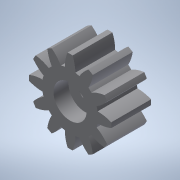
# Autodesk Inventor part: small-gear
Saved by Autodesk Inventor 2020 (Build 240168000, 168)
## iProperties
Created: 2020-05-22
Part Number: small-gear
Material: Ogólny
Document SubType Name: Modeling
Designer: blep
Density: 1 g/cm^3
Appearance: Domyślna
Author: blep
Autodesk Inventor part; units mm, degrees
ref_plane "YZ Plane" through (0, 0, 0) normal (1, 0, 0) x (0, 1, 0)
ref_plane "XZ Plane" through (0, 0, 0) normal (0, 1, 0) x (-1, 0, 0)
ref_plane "XY Plane" through (0, 0, 0) normal (0, 0, 1) x (1, 0, 0)
sketch "Szkic1" plane through (0, 0, 0) normal (0, 0, 1) x (1, 0, 0)
  arc A0 (-1.732, -4.0613) -> (-1.6613, -4.132) centre (0, -2.4) ccw projected
  arc A1 (0.05, -0.4006) -> (-0.05, -0.4006) centre (0, -2.4) ccw projected
  arc A2 (-0.05, -0.4006) -> (-0.5703, -0.483) centre (0, -2.4) ccw projected
  arc A3 (-0.5703, -0.483) -> (-0.6654, -0.5139) centre (0, -2.4) ccw projected
  arc A4 (-0.6654, -0.5139) -> (-1.1348, -0.7531) centre (0, -2.4) ccw projected
  arc A5 (-1.1348, -0.7531) -> (-1.2157, -0.8119) centre (0, -2.4) ccw projected
  arc A6 (-1.2157, -0.8119) -> (-1.5881, -1.1843) centre (0, -2.4) ccw projected
  arc A7 (-1.5881, -1.1843) -> (-1.6469, -1.2652) centre (0, -2.4) ccw projected
  arc A8 (-1.6469, -1.2652) -> (-1.8861, -1.7346) centre (0, -2.4) ccw projected
  arc A9 (-1.8861, -1.7346) -> (-1.917, -1.8297) centre (0, -2.4) ccw projected
  arc A10 (-1.917, -1.8297) -> (-1.9994, -2.35) centre (0, -2.4) ccw projected
  arc A11 (-1.9994, -2.35) -> (-1.9994, -2.45) centre (0, -2.4) ccw projected
  arc A12 (-1.9994, -2.45) -> (-1.917, -2.9703) centre (0, -2.4) ccw projected
  arc A13 (-1.917, -2.9703) -> (-1.8861, -3.0654) centre (0, -2.4) ccw projected
  arc A14 (-1.8861, -3.0654) -> (-1.6469, -3.5348) centre (0, -2.4) ccw projected
  arc A15 (-1.6469, -3.5348) -> (-1.5881, -3.6157) centre (0, -2.4) ccw projected
  arc A16 (-1.5881, -3.6157) -> (-1.2157, -3.9881) centre (0, -2.4) ccw projected
  arc A17 (-1.2157, -3.9881) -> (-1.1348, -4.0469) centre (0, -2.4) ccw projected
  arc A18 (-1.1348, -4.0469) -> (-0.6654, -4.2861) centre (0, -2.4) ccw projected
  arc A19 (-0.6654, -4.2861) -> (-0.5703, -4.317) centre (0, -2.4) ccw projected
  arc A20 (-0.5703, -4.317) -> (-0.05, -4.3994) centre (0, -2.4) ccw projected
  arc A21 (-0.05, -4.3994) -> (0.05, -4.3994) centre (0, -2.4) ccw projected
  arc A22 (0.05, -4.3994) -> (0.5703, -4.317) centre (0, -2.4) ccw projected
  arc A23 (0.5703, -4.317) -> (0.6654, -4.2861) centre (0, -2.4) ccw projected
  arc A24 (0.6654, -4.2861) -> (1.1348, -4.0469) centre (0, -2.4) ccw projected
  arc A25 (1.1348, -4.0469) -> (1.2157, -3.9881) centre (0, -2.4) ccw projected
  arc A26 (1.2157, -3.9881) -> (1.5881, -3.6157) centre (0, -2.4) ccw projected
  arc A27 (1.5881, -3.6157) -> (1.6469, -3.5348) centre (0, -2.4) ccw projected
  arc A28 (1.6469, -3.5348) -> (1.8861, -3.0654) centre (0, -2.4) ccw projected
  arc A29 (1.8861, -3.0654) -> (1.917, -2.9703) centre (0, -2.4) ccw projected
  arc A30 (1.917, -2.9703) -> (1.9994, -2.45) centre (0, -2.4) ccw projected
  arc A31 (1.9994, -2.45) -> (1.9994, -2.35) centre (0, -2.4) ccw projected
  arc A32 (1.9994, -2.35) -> (1.917, -1.8297) centre (0, -2.4) ccw projected
  arc A33 (1.917, -1.8297) -> (1.8861, -1.7346) centre (0, -2.4) ccw projected
  arc A34 (1.8861, -1.7346) -> (1.6469, -1.2652) centre (0, -2.4) ccw projected
  arc A35 (1.6469, -1.2652) -> (1.5881, -1.1843) centre (0, -2.4) ccw projected
  arc A36 (1.5881, -1.1843) -> (1.2157, -0.8119) centre (0, -2.4) ccw projected
  arc A37 (1.2157, -0.8119) -> (1.1348, -0.7531) centre (0, -2.4) ccw projected
  arc A38 (1.1348, -0.7531) -> (0.6654, -0.5139) centre (0, -2.4) ccw projected
  arc A39 (0.6654, -0.5139) -> (0.5703, -0.483) centre (0, -2.4) ccw projected
  arc A40 (0.5703, -0.483) -> (0.05, -0.4006) centre (0, -2.4) ccw projected
  circle A41 centre (0, -2.4) radius 1.5065 projected
  circle A42 centre (0, -2.4) radius 2.4
  circle A43 centre (0, -2.4) radius 15
  circle A44 centre (0, -2.4) radius 1.0065 projected
  circle A45 centre (0, -2.4) radius 1.2565
  circle A46 centre (0, -2.4) radius 2.65
  point P0 (0, 0)
  point P1 (-1.6613, -4.132)
  point P2 (-1.732, -4.0613)
  dimension "d0" = 30
  dimension "d3" = 0.25
  dimension "d12" = 0.25
  constraints: 4 centre point, 2 coincident, 1 concentric
  measures "d0" diameter of A43
  measures "d3" radial gap between concentric circles of A44 A45
  measures "d12" radial gap between concentric circles of A42 A46
extrude "Wyciągnięcie proste1" add sketch "Szkic1" against normal blind 3 contours A43
extrude "Wyciągnięcie proste2" add sketch "Szkic1" along normal blind 1.5 contours A42 A0 | A40 A39 A38 A37 A36 A35 A34 A33 A32 A31 A30 A29 A28 A27 A26 A25 A24 A23 A22 A21 A20 A19 A18 A17 A16 A15 A14 A13 A12 A11 A10 A9 A8 A7 A6 A5 A4 A3 A2 A1 | A41 | A43 | A45 | A46
sketch "Szkic2" plane through (0, -2.4, 1.5) normal (0, 0, 1) x (1, 0, 0)
  circle A0 centre (0, 0) radius 1.0065 projected
  circle A1 centre (0, 0) radius 3
  circle A2 centre (0, 0) radius 15 projected
  point P0 (0, 2.4)
  dimension "d6" = 6
  constraints: 1 centre point, 1 coincident
  measures "d6" diameter of A1
extrude "Wyciągnięcie proste3" add sketch "Szkic2" along normal blind 2.7 contours A2
spur gear teeth "Przekładnia walcowa1" teeth 12 pitch diameter 13.5 tip diameter 15.0027 root diameter 10.2375 face width 7.6 trims to tip circle yes start plane through (0, -2.4, -3) normal (0, 0, -1) x (-1, 0, 0)
sketch "Szkic3" plane through (0, -2.4, 4.2) normal (0, 0, 1) x (1, 0, 0)
  arc A0 (-6.2371, 4.1675) -> (-6.7277, 3.3178) centre (0, 0) ccw projected
  arc A1 (-6.7277, 3.3178) -> (-4.8471, 1.6454) centre (-1.5303, 7.2689) ccw projected
  arc A2 (-4.8471, 1.6454) -> (-5.0204, 0.9986) centre (0, 0) ccw projected
  arc A3 (-5.0204, 0.9986) -> (-7.4853, 0.4906) centre (-4.9597, -5.5299) ccw projected
  arc A4 (-7.4853, 0.4906) -> (-7.4853, -0.4906) centre (0, 0) ccw projected
  arc A5 (-7.4853, -0.4906) -> (-5.0204, -0.9986) centre (-4.9597, 5.5299) ccw projected
  arc A6 (-5.0204, -0.9986) -> (-4.8471, -1.6454) centre (0, 0) ccw projected
  arc A7 (-4.8471, -1.6454) -> (-6.7277, -3.3178) centre (-1.5303, -7.2689) ccw projected
  arc A8 (-6.7277, -3.3178) -> (-6.2371, -4.1675) centre (0, 0) ccw projected
  arc A9 (-6.2371, -4.1675) -> (-3.8485, -3.375) centre (-7.0601, 2.3092) ccw projected
  arc A10 (-3.8485, -3.375) -> (-3.375, -3.8485) centre (0, 0) ccw projected
  arc A11 (-3.375, -3.8485) -> (-4.1675, -6.2371) centre (2.3092, -7.0601) ccw projected
  arc A12 (-4.1675, -6.2371) -> (-3.3178, -6.7277) centre (0, 0) ccw projected
  arc A13 (-3.3178, -6.7277) -> (-1.6454, -4.8471) centre (-7.2689, -1.5303) ccw projected
  arc A14 (-1.6454, -4.8471) -> (-0.9986, -5.0204) centre (0, 0) ccw projected
  arc A15 (-0.9986, -5.0204) -> (-0.4906, -7.4853) centre (5.5299, -4.9597) ccw projected
  arc A16 (-0.4906, -7.4853) -> (0.4906, -7.4853) centre (0, 0) ccw projected
  arc A17 (0.4906, -7.4853) -> (0.9986, -5.0204) centre (-5.5299, -4.9597) ccw projected
  arc A18 (0.9986, -5.0204) -> (1.6454, -4.8471) centre (0, 0) ccw projected
  arc A19 (1.6454, -4.8471) -> (3.3178, -6.7277) centre (7.2689, -1.5303) ccw projected
  arc A20 (3.3178, -6.7277) -> (4.1675, -6.2371) centre (0, 0) ccw projected
  arc A21 (4.1675, -6.2371) -> (3.375, -3.8485) centre (-2.3092, -7.0601) ccw projected
  arc A22 (3.375, -3.8485) -> (3.8485, -3.375) centre (0, 0) ccw projected
  arc A23 (3.8485, -3.375) -> (6.2371, -4.1675) centre (7.0601, 2.3092) ccw projected
  arc A24 (6.2371, -4.1675) -> (6.7277, -3.3178) centre (0, 0) ccw projected
  arc A25 (6.7277, -3.3178) -> (4.8471, -1.6454) centre (1.5303, -7.2689) ccw projected
  arc A26 (4.8471, -1.6454) -> (5.0204, -0.9986) centre (0, 0) ccw projected
  arc A27 (5.0204, -0.9986) -> (7.4853, -0.4906) centre (4.9597, 5.5299) ccw projected
  arc A28 (7.4853, -0.4906) -> (7.4853, 0.4906) centre (0, 0) ccw projected
  arc A29 (7.4853, 0.4906) -> (5.0204, 0.9986) centre (4.9597, -5.5299) ccw projected
  arc A30 (5.0204, 0.9986) -> (4.8471, 1.6454) centre (0, 0) ccw projected
  arc A31 (4.8471, 1.6454) -> (6.7277, 3.3178) centre (1.5303, 7.2689) ccw projected
  arc A32 (6.7277, 3.3178) -> (6.2371, 4.1675) centre (0, 0) ccw projected
  arc A33 (6.2371, 4.1675) -> (3.8485, 3.375) centre (7.0601, -2.3092) ccw projected
  arc A34 (3.8485, 3.375) -> (3.375, 3.8485) centre (0, 0) ccw projected
  arc A35 (3.375, 3.8485) -> (4.1675, 6.2371) centre (-2.3092, 7.0601) ccw projected
  arc A36 (4.1675, 6.2371) -> (3.3178, 6.7277) centre (0, 0) ccw projected
  arc A37 (3.3178, 6.7277) -> (1.6454, 4.8471) centre (7.2689, 1.5303) ccw projected
  arc A38 (1.6454, 4.8471) -> (0.9986, 5.0204) centre (0, 0) ccw projected
  arc A39 (0.9986, 5.0204) -> (0.4906, 7.4853) centre (-5.5299, 4.9597) ccw projected
  arc A40 (0.4906, 7.4853) -> (-0.4906, 7.4853) centre (0, 0) ccw projected
  arc A41 (-0.4906, 7.4853) -> (-0.9986, 5.0204) centre (5.5299, 4.9597) ccw projected
  arc A42 (-0.9986, 5.0204) -> (-1.6454, 4.8471) centre (0, 0) ccw projected
  arc A43 (-1.6454, 4.8471) -> (-3.3178, 6.7277) centre (-7.2689, 1.5303) ccw projected
  arc A44 (-3.3178, 6.7277) -> (-4.1675, 6.2371) centre (0, 0) ccw projected
  arc A45 (-4.1675, 6.2371) -> (-3.375, 3.8485) centre (2.3092, 7.0601) ccw projected
  arc A46 (-3.375, 3.8485) -> (-3.8485, 3.375) centre (0, 0) ccw projected
  arc A47 (-3.8485, 3.375) -> (-6.2371, 4.1675) centre (-7.0601, -2.3092) ccw projected
  circle A48 centre (0, 0) radius 3 projected
  arc A49 (4.1139, -6.2127) -> (3.3113, -3.8376) centre (-2.3092, -7.0601) ccw
  arc A50 (3.3234, -6.6691) -> (4.1139, -6.2127) centre (0, 0) ccw
  arc A51 (1.6678, -4.7865) -> (3.3234, -6.6691) centre (7.2689, -1.5303) ccw
  arc A52 (0.9489, -4.9791) -> (1.6678, -4.7865) centre (0, 0) ccw
  arc A53 (0.4564, -7.4373) -> (0.9489, -4.9791) centre (-5.5299, -4.9597) ccw
  arc A54 (-0.4564, -7.4373) -> (0.4564, -7.4373) centre (0, 0) ccw
  arc A55 (-0.9489, -4.9791) -> (-0.4564, -7.4373) centre (5.5299, -4.9597) ccw
  arc A56 (-1.6678, -4.7865) -> (-0.9489, -4.9791) centre (0, 0) ccw
  arc A57 (-3.3234, -6.6691) -> (-1.6678, -4.7865) centre (-7.2689, -1.5303) ccw
  arc A58 (-4.1139, -6.2127) -> (-3.3234, -6.6691) centre (0, 0) ccw
  arc A59 (-3.3113, -3.8376) -> (-4.1139, -6.2127) centre (2.3092, -7.0601) ccw
  arc A60 (-3.8376, -3.3113) -> (-3.3113, -3.8376) centre (0, 0) ccw
  arc A61 (-6.2127, -4.1139) -> (-3.8376, -3.3113) centre (-7.0601, 2.3092) ccw
  arc A62 (-6.6691, -3.3234) -> (-6.2127, -4.1139) centre (0, 0) ccw
  arc A63 (-4.7865, -1.6678) -> (-6.6691, -3.3234) centre (-1.5303, -7.2689) ccw
  arc A64 (-4.9791, -0.9489) -> (-4.7865, -1.6678) centre (0, 0) ccw
  arc A65 (-7.4373, -0.4564) -> (-4.9791, -0.9489) centre (-4.9597, 5.5299) ccw
  arc A66 (-7.4373, 0.4564) -> (-7.4373, -0.4564) centre (0, 0) ccw
  arc A67 (-4.9791, 0.9489) -> (-7.4373, 0.4564) centre (-4.9597, -5.5299) ccw
  arc A68 (-4.7865, 1.6678) -> (-4.9791, 0.9489) centre (0, 0) ccw
  arc A69 (-6.6691, 3.3234) -> (-4.7865, 1.6678) centre (-1.5303, 7.2689) ccw
  arc A70 (-6.2127, 4.1139) -> (-6.6691, 3.3234) centre (0, 0) ccw
  arc A71 (-3.8376, 3.3113) -> (-6.2127, 4.1139) centre (-7.0601, -2.3092) ccw
  arc A72 (-3.3113, 3.8376) -> (-3.8376, 3.3113) centre (0, 0) ccw
  arc A73 (-4.1139, 6.2127) -> (-3.3113, 3.8376) centre (2.3092, 7.0601) ccw
  arc A74 (-3.3234, 6.6691) -> (-4.1139, 6.2127) centre (0, 0) ccw
  arc A75 (-1.6678, 4.7865) -> (-3.3234, 6.6691) centre (-7.2689, 1.5303) ccw
  arc A76 (-0.9489, 4.9791) -> (-1.6678, 4.7865) centre (0, 0) ccw
  arc A77 (-0.4564, 7.4373) -> (-0.9489, 4.9791) centre (5.5299, 4.9597) ccw
  arc A78 (0.4564, 7.4373) -> (-0.4564, 7.4373) centre (0, 0) ccw
  arc A79 (0.9489, 4.9791) -> (0.4564, 7.4373) centre (-5.5299, 4.9597) ccw
  arc A80 (1.6678, 4.7865) -> (0.9489, 4.9791) centre (0, 0) ccw
  arc A81 (3.3234, 6.6691) -> (1.6678, 4.7865) centre (7.2689, 1.5303) ccw
  arc A82 (4.1139, 6.2127) -> (3.3234, 6.6691) centre (0, 0) ccw
  arc A83 (3.3113, 3.8376) -> (4.1139, 6.2127) centre (-2.3092, 7.0601) ccw
  arc A84 (3.8376, 3.3113) -> (3.3113, 3.8376) centre (0, 0) ccw
  arc A85 (6.2127, 4.1139) -> (3.8376, 3.3113) centre (7.0601, -2.3092) ccw
  arc A86 (6.6691, 3.3234) -> (6.2127, 4.1139) centre (0, 0) ccw
  arc A87 (4.7865, 1.6678) -> (6.6691, 3.3234) centre (1.5303, 7.2689) ccw
  arc A88 (4.9791, 0.9489) -> (4.7865, 1.6678) centre (0, 0) ccw
  arc A89 (7.4373, 0.4564) -> (4.9791, 0.9489) centre (4.9597, -5.5299) ccw
  arc A90 (7.4373, -0.4564) -> (7.4373, 0.4564) centre (0, 0) ccw
  arc A91 (4.9791, -0.9489) -> (7.4373, -0.4564) centre (4.9597, 5.5299) ccw
  arc A92 (4.7865, -1.6678) -> (4.9791, -0.9489) centre (0, 0) ccw
  arc A93 (6.6691, -3.3234) -> (4.7865, -1.6678) centre (1.5303, -7.2689) ccw
  arc A94 (6.2127, -4.1139) -> (6.6691, -3.3234) centre (0, 0) ccw
  arc A95 (3.8376, -3.3113) -> (6.2127, -4.1139) centre (7.0601, 2.3092) ccw
  arc A96 (3.3113, -3.8376) -> (3.8376, -3.3113) centre (0, 0) ccw
  point P0 (0, 2.4)
  dimension "d9" = 0.05
  constraints: 96 point on circle, 48 centre point, 47 other
  measures "d9" radial gap between concentric circles of A21 A49
extrude "Wyciągnięcie proste4" cut sketch "Szkic3" against normal through all contours A47 A46 A45 A44 A43 A42 A41 A40 A39 A38 A37 A36 A35 A34 A33 A32 A31 A30 A29 A28 A27 A26 A25 A24 A23 A22 A21 A20 A19 A18 A17 A16 A15 A14 A13 A12 A11 A10 A9 A8 A7 A6 A5 A4 A3 A2 A1 A0
